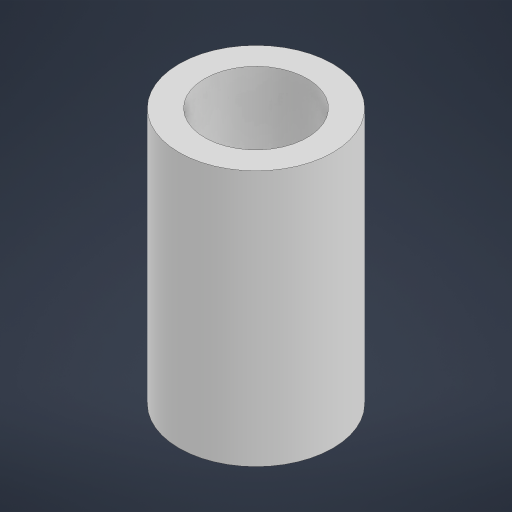
# Autodesk Inventor part: base
Saved by Autodesk Inventor 2024.3 (Build 283343000, 343)
## iProperties
Created: 2024-09-28
Part Number: base
Material: Generic
Document SubType Name: Modeling
Designer: sam
Density: 1 g/cm^3
Appearance: Default
Sheet Metal Rule: Default
Author: sam
Autodesk Inventor part; units mm, degrees
ref_plane "YZ Plane" through (0, 0, 0) normal (1, 0, 0) x (0, 1, 0)
ref_plane "XZ Plane" through (0, 0, 0) normal (0, 1, 0) x (-1, 0, 0)
ref_plane "XY Plane" through (0, 0, 0) normal (0, 0, 1) x (1, 0, 0)
sketch "Sketch1" plane through (0, 0, 0) normal (0, 1, 0) x (-1, 0, 0)
  line L0 (3.5364, -1.5) -> (3.5, -1.5)
  line L1 (1.5, 3.5) -> (1.5, 3.5)
  line L2 (3.5, 1.5) -> (3.5, 1.5)
  line L3 (-1.5, 3.5) -> (-1.5, 3.5364)
  line L4 (-1.5, -1.5) -> (1.5, 1.5) construction
  line L5 (1.5, -1.5) -> (-1.5, 1.5) construction
  circle A0 centre (0, 0) radius 1
  line L6 (0, 1.5) -> (0, 1.5)
  line L7 (1.5, 0) -> (1.5, 0)
  line L8 (0, -1.5) -> (0, -1.5)
  line L9 (-1.5, 0) -> (-1.5, 0)
  arc A1 (0, 1.5) -> (-1.5, 0) centre (0, 0) ccw
  arc A2 (-1.5, 0) -> (0, -1.5) centre (0, 0) ccw
  arc A3 (0, -1.5) -> (1.5, 0) centre (0, 0) ccw
  arc A4 (1.5, 0) -> (0, 1.5) centre (0, 0) ccw
  point P0 (-1.5, 0)
  dimension "d46" = 2
  dimension "d48" = 3
  dimension "d49" = 3
  dimension "d50" = 1.5
  constraints: 20 end point, 12 point on line, 8 point on circle, 8 tangent, 5 centre point, 4 parallel, 3 concentric, 2 horizontal, 2 midpoint, 2 perpendicular, 1 coincident
  measures "d46" diameter of A0
  measures "d48" distance between parallel lines of L8 L6
  measures "d49" distance between parallel lines of L9 L7
  measures "d50" radius of A1
extrude "Extrusion1" add sketch "Sketch1" along normal blind 5
equation "\"BendRadius\" = Thickness"
equation "\"BendReliefWidth\" = Thickness"
equation "\"BendReliefDepth\" = 0.5 * Thickness"
equation "\"CornerReliefSize\" = 4 * Thickness"
equation "\"MinimumRemnant\" = 2 * Thickness"
equation "\"TransitionRadius\" = BendRadius"
equation "\"JacobiRadiusSize\" = BendRadius"
equation "\"GapSize\" = Thickness"
equation "\"Thickness\" = 3.048"
body "Solid1"
